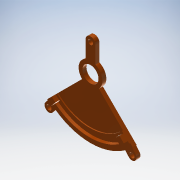
# Autodesk Inventor part: Yaw Platform Top
Saved by Autodesk Inventor 2018.2 (Build 222227000, 227)
## iProperties
Created: 2018-02-12
Part Number: Yaw Platform Top
Material: ABS Plastic
Document SubType Name: Modeling
Designer: Moochster
Density: 1.06 g/cm^3
Appearance: Smooth - Light Orange
Author: Moochster
Autodesk Inventor part; units mm, degrees
ref_plane "YZ Plane" through (0, 0, 0) normal (1, 0, 0) x (0, 1, 0)
ref_plane "XZ Plane" through (0, 0, 0) normal (0, 1, 0) x (-1, 0, 0)
ref_plane "XY Plane" through (0, 0, 0) normal (0, 0, 1) x (1, 0, 0)
sketch "Sketch1" plane through (0, 0, 0) normal (0, 1, 0) x (-1, 0, 0)
  circle A0 centre (0, 0) radius 7.9375 construction
  circle A1 centre (0, 0) radius 8.0875
  circle A2 centre (0, 28) radius 2.5
  line L0 (0, 0) -> (0, 28) construction
  arc A3 (-42.426407, -42.426407) -> (42.426407, -42.426407) centre (0, 0) ccw
  circle A4 centre (0, 0) radius 11.9375
  line L1 (42.426407, -42.426407) -> (8.441087, -8.441087)
  line L2 (-42.426407, -42.426407) -> (-8.441087, -8.441087)
  line L3 (5, 10.839922) -> (5, 28)
  arc A5 (5, 28) -> (-5, 28) centre (0, 28) ccw
  line L4 (-5, 28) -> (-5, 10.839922)
  dimension "d0" = 15.875
  dimension "d1" = 0.15
  dimension "d2" = 5
  dimension "d5" = 28
  dimension "d8" = 4
  dimension "d11" = 90
  dimension "d12" = 60
  dimension "d13" = 10
  constraints: 10 end point, 8 point on circle, 6 centre point, 3 coincident, 2 concentric, 2 point on line, 2 tangent, 2 vertical, 1 parallel, 1 vertical alignment, 1 other
  measures "d0" diameter of A0
  measures "d1" radial gap between concentric circles of A0 A1
  measures "d2" diameter of A2
  measures "d5" distance of L0.start L0.end
  measures "d8" radial gap between concentric circles of A4 A0
  measures "d11" angle of L2 L1
  measures "d12" radius of A3
  measures "d13" distance between parallel lines of L4 L3
extrude "Extrusion1" add sketch "Sketch1" along normal blind 4
sketch "Sketch2" plane through (42.426407, 0, -42.426407) normal (0.7071068, 0, 0.7071068) x (0.7071068, 0, -0.7071068)
  line L0 (0, 0) -> (-60, 0)
  line L1 (-3.5, 0) -> (-3.5, -1)
  line L2 (-3.5, -1) -> (-5.5, -1)
  line L3 (-5.5, -1) -> (-6.169873, 1.5)
  line L4 (-6.169873, 1.5) -> (-11.169873, 1.5)
  line L5 (-11.169873, 1.5) -> (-11.839746, -1)
  line L6 (-11.839746, -1) -> (-13.839746, -1)
  line L7 (-3.5, 0) -> (-5.767949, 0)
  line L8 (-11.571797, 0) -> (-13.839746, 0)
  line L9 (-13.839746, -1) -> (-13.839746, 0)
  line L10 (0, 0) -> (0, 4)
  dimension "d14" = 1
  dimension "d15" = 5
  dimension "d16" = 1.5
  dimension "d17" = 15
  dimension "d18" = 2
  dimension "d19" = 3.5
  constraints: 18 end point, 6 point on line, 2 equal length, 2 perpendicular, 1 collinear, 1 horizontal alignment, 1 parallel, 1 vertical
  measures "d14" distance of L1.start L1.end
  measures "d15" distance of L3.end L4.end
  measures "d16" distance between parallel lines of L0 L4
  measures "d17" angle of L9 L5
  measures "d18" distance of L1.end L2.end
  measures "d19" distance between parallel lines of L10 L1
sketch3d "3D Sketch1"
  arc A0 (42.426407, 0, -42.426407) -> (-42.426407, 0, -42.426407) centre (0, 0, 0) ccw
sweep "Sweep1" add profiles "Sketch2" path "3D Sketch1" contours L1 L2 L3 L0 | L5 L6 L9 L0
sketch3d "3D Sketch2"
  arc A0 (38.347851, 0, -38.347851) -> (-38.347851, 0, -38.347851) centre (0, 0, 0) ccw
sweep "Sweep2" cut profiles "Sketch2" path "3D Sketch2" contours L0 L5 L4 L3
sketch "Sketch3" plane through (0, 4, 0) normal (0, 1, 0) x (1, 0, 0)
  circle A0 centre (0, -28) radius 2.5
  circle A1 centre (0, 0) radius 8.0875
  arc A2 (5, -10.839922) -> (8.441087, 8.441087) centre (0, 0) ccw
  line L0 (8.441087, 8.441087) -> (42.426407, 42.426407)
  arc A3 (42.426407, 42.426407) -> (-42.426407, 42.426407) centre (0, 0) ccw
  line L1 (-42.426407, 42.426407) -> (-8.441087, 8.441087)
  arc A4 (-8.441087, 8.441087) -> (-5, -10.839922) centre (0, 0) ccw
  line L2 (-5, -10.839922) -> (-5, -28)
  arc A5 (-5, -28) -> (5, -28) centre (0, -28) ccw
  line L3 (5, -28) -> (5, -10.839922)
  circle A6 centre (41.781195, 49.792889) radius 2.5
  arc A7 (45.228395, 46.900345) -> (38.333995, 52.685433) centre (41.781195, 49.792889) ccw
  line L4 (38.333995, 52.685433) -> (35.011433, 48.725759)
  arc A8 (42.426407, 42.426407) -> (-42.426407, 42.426407) centre (0, 0) ccw
  line L5 (8.441087, 8.441087) -> (42.426407, 42.426407)
  line L6 (45.228395, 46.900345) -> (41.905833, 42.94067)
  line L7 (41.781195, 49.792889) -> (0, 0) construction
  line L8 (0, 0) -> (0, 73.873474) construction
  dimension "d24" = 5
  dimension "d25" = 2
  dimension "d33" = 40
  dimension "d34" = 65
  constraints: 8 end point, 4 point on circle, 2 centre point, 2 parallel, 2 tangent, 1 concentric, 1 vertical
  measures "d24" diameter of A6
  measures "d25" radial gap between concentric circles of A7 A6
  measures "d33" angle of L7 L8
  measures "d34" distance of L7.start L7.end
extrude "Extrusion2" add sketch "Sketch3" against normal up to surface (4 mm away) contours A3 L4 A7 L6
mirror "Mirror1" about plane through (0, 0, 0) normal (1, 0, 0) of "Extrusion2"
sketch "Sketch4" plane through (8.441087, 0, -8.441087) normal (0.7071068, 0, 0.7071068) x (0.7071068, 0, -0.7071068)
  line L0 (36.222754, -1) -> (36.892627, 1.5)
  line L1 (36.892627, 1.5) -> (41.892627, 1.5)
  line L2 (41.892627, 1.5) -> (42.5625, -1)
  line L3 (42.5625, -1) -> (42.5625, -5)
  line L4 (42.5625, -5) -> (36.222754, -5)
  line L5 (36.222754, -5) -> (36.222754, -1)
  point P0 (-11.9375, 0)
  dimension "d29" = 4
  constraints: 6 end point, 2 perpendicular, 1 vertical
  measures "d29" distance of L2.end L3.end
sketch "Sketch5" plane through (0, 1.5, 0) normal (0, -1, 0) x (1, 0, 0)
  arc A0 (30.816205, -37.877999) -> (34.528114, -34.528114) centre (0, 0) ccw
  arc A1 (-34.528114, -34.528114) -> (34.528114, -34.528114) centre (0, 0) ccw construction
  point P0 (0, 0)
  dimension "d30" = 5
  constraints: 3 point on circle, 1 centre point, 1 coincident, 1 concentric
  measures "d30" distance of A0.end A0.start
sweep "Sweep3" add profiles "Sketch4" path "Sketch5"
mirror "Mirror2" about plane through (0, 0, 0) normal (1, 0, 0) of "Sweep3"
body "Solid1"
